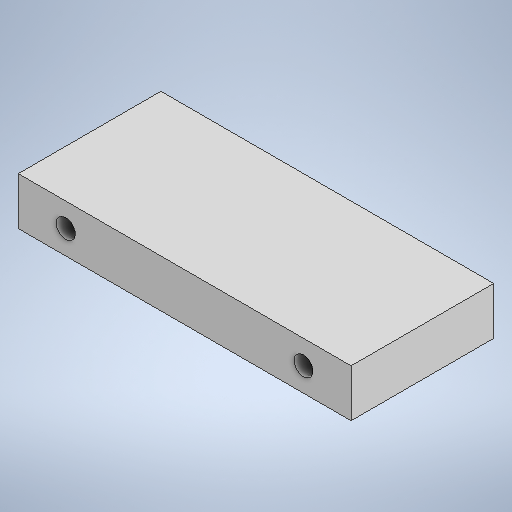
# Autodesk Inventor part: Schiebegewicht Wand
Saved by Autodesk Inventor 2025 (Build 290162000, 162)
## iProperties
Created: 2026-01-07
Part Number: Schiebegewicht Wand
Material: Generic
Document SubType Name: Modeling
Designer: ruven
Density: 1 g/cm^3
Appearance: Default
Author: ruven
Autodesk Inventor part; units mm, degrees
ref_plane "YZ Plane" through (0, 0, 0) normal (1, 0, 0) x (0, 1, 0)
ref_plane "XZ Plane" through (0, 0, 0) normal (0, 1, 0) x (-1, 0, 0)
ref_plane "XY Plane" through (0, 0, 0) normal (0, 0, 1) x (1, 0, 0)
sketch "Sketch1" plane through (0, 0, 0) normal (0, 1, 0) x (-1, 0, 0)
  line L0 (33.2073, 5) -> (-36.7927, 5)
  line L1 (-36.7927, 5) -> (-36.7927, -5)
  line L2 (-36.7927, -5) -> (33.2073, -5)
  line L3 (33.2073, -5) -> (33.2073, 5)
  line L4 (33.2073, 5) -> (-36.7927, -5) construction
  line L5 (-36.7927, 5) -> (33.2073, -5) construction
  circle A0 centre (23.2073, 0) radius 2
  circle A1 centre (-26.7927, 0) radius 2
  point P0 (-1.7927, 0)
  point P1 (-1.7927, -5)
  dimension "d0" = 10
  dimension "d4" = 70
  dimension "d5" = 4
  dimension "d6" = 4
  dimension "d7" = 10
  dimension "d8" = 10
  dimension "d9" = 50
  constraints: 12 end point, 3 midpoint, 2 centre point, 2 parallel, 1 horizontal, 1 perpendicular
  measures "d0" distance between parallel lines of L2 L0
  measures "d4" distance of L0.start L0.end
  measures "d5" diameter of A0
  measures "d6" diameter of A1
  measures "d7" distance from line of L1 A1.centre
  measures "d8" distance from line of L3 A0.centre
  measures "d9" distance of A1.centre A0.centre
extrude "Extrusion1" add sketch "Sketch1" along normal blind 30
body "Solid1"
